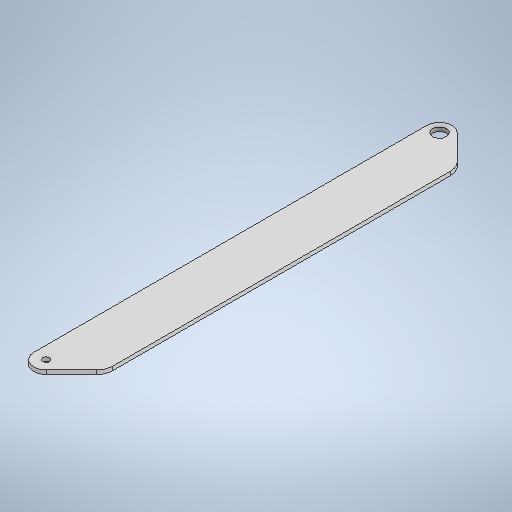
# Autodesk Inventor part: A2P4
Saved by Autodesk Inventor 2025.2 (Build 292293000, 293)
## iProperties
Created: 2025-05-22
Part Number: A2P4
Material: Generic
Document SubType Name: Modeling
Designer: Verchasv
Density: 1 g/cm^3
Appearance: Default
Author: Verchasv
Autodesk Inventor part; units mm, degrees
ref_plane "YZ Plane" through (0, 0, 0) normal (1, 0, 0) x (0, 1, 0)
ref_plane "XZ Plane" through (0, 0, 0) normal (0, 1, 0) x (-1, 0, 0)
ref_plane "XY Plane" through (0, 0, 0) normal (0, 0, 1) x (1, 0, 0)
sketch "Sketch1" plane through (0, 0, 0) normal (0, 1, 0) x (-1, 0, 0)
  arc A0 (7.808, 86.5621) -> (-1.4957, 90.4158) centre (2.358, 86.5621) ccw
  line L0 (7.808, 86.5621) -> (7.808, -83.4379)
  line L1 (-1.4957, 90.4158) -> (-12.3494, 79.5621)
  arc A1 (-12.3494, 79.5621) -> (-14.4205, 74.5621) centre (-7.3494, 74.5621) ccw
  line L2 (-14.4205, 74.5621) -> (-14.4205, -71.4379)
  arc A2 (-1.4957, -87.2917) -> (7.808, -83.4379) centre (2.358, -83.4379) ccw
  line L3 (-1.4957, -87.2917) -> (-12.3494, -76.4379)
  arc A3 (-14.4205, -71.4379) -> (-12.3494, -76.4379) centre (-7.3494, -71.4379) ccw
  point P0 (0, 0)
  dimension "d0" = 10.9
  dimension "d1" = 170
  dimension "d2" = 0
  dimension "d3" = 12
  dimension "d4" = 12
  dimension "d5" = 5.45
  dimension "d6" = 45
  dimension "d7" = 7
  dimension "d8" = 7
  dimension "d9" = 10.9
  dimension "d10" = 135
  constraints: 8 end point, 8 point on circle, 5 tangent, 4 centre point, 2 vertical, 1 coincident
  measures "d0" diameter of A0
  measures "d1" distance of A2.centre point (2.358, 86.562)
  measures "d2" horizontal distance of A2.centre point (2.358, 86.562)
  measures "d3" vertical distance of L2.start point (2.358, 86.562)
  measures "d4" vertical distance of L2.end A2.centre
  measures "d5" distance from line of point (2.358, 86.562) L0
  measures "d6" angle of L0 L1
  measures "d7" vertical distance of point (2.358, 86.562) L1.end
  measures "d8" vertical distance of A2.centre L3.end
  measures "d9" diameter of A2
  measures "d10" angle of L3 L0
extrude "Extrusion1" add sketch "Sketch1" along normal blind 1.7
sketch "Sketch2" plane through (0, 1.7, 0) normal (0, 1, 0) x (1, 0, 0)
  arc A0 (1.4957, 87.2917) -> (-7.808, 83.4379) centre (-2.358, 83.4379) ccw projected
  arc A1 (-7.808, -86.5621) -> (1.4957, -90.4158) centre (-2.358, -86.5621) ccw projected
  circle A2 centre (-2.358, 83.4379) radius 3
  circle A3 centre (-2.358, -86.5621) radius 1.5
  point P0 (0, 0)
  dimension "d13" = 6
  dimension "d14" = 3
  constraints: 2 centre point, 2 coincident
  measures "d13" diameter of A2
  measures "d14" diameter of A3
extrude "Extrusion2" cut sketch "Sketch2" against normal through all
body "Solid1"
